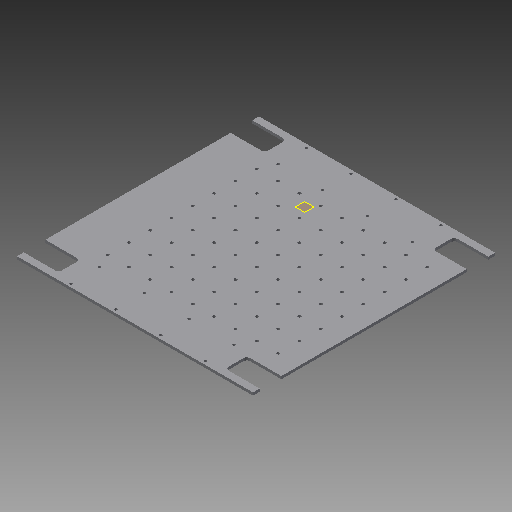
# Autodesk Inventor part: 1021TopP
Saved by Autodesk Inventor 2017 (Build 210142000, 142)
## iProperties
Created: 2016-09-29
Part Number: 1021TopP
Material: Generic
Document SubType Name: Modeling
Designer: Adam Popescu
Density: 1 g/cm^3
Appearance: Default
Author: Adam Popescu
Autodesk Inventor part; units mm, degrees
ref_plane "YZ Plane" through (0, 0, 0) normal (1, 0, 0) x (0, 1, 0)
ref_plane "XZ Plane" through (0, 0, 0) normal (0, 1, 0) x (-1, 0, 0)
ref_plane "XY Plane" through (0, 0, 0) normal (0, 0, 1) x (1, 0, 0)
sketch "Sketch1" plane through (0, 0, 0) normal (0, 1, 0) x (-1, 0, 0)
  circle A0 centre (-196.9946, -55.8186) radius 3.175
  circle A1 centre (-196.9946, -122.4936) radius 3.175
  circle A2 centre (-91.9021, -55.8186) radius 3.175
  circle A3 centre (13.1904, -55.8186) radius 3.175
  circle A4 centre (118.2829, -55.8186) radius 3.175
  circle A5 centre (-91.9021, -122.4936) radius 3.175
  circle A6 centre (13.1904, -122.4936) radius 3.175
  circle A7 centre (118.2829, -122.4936) radius 3.175
  line L0 (1428.2628, 61.5049) -> (1440.9628, 61.5049)
  line L1 (1966.4253, 57.5049) -> (1979.1253, 57.5049)
  circle A8 centre (-196.9946, 429.6364) radius 3.175
  circle A9 centre (-196.9946, 362.9614) radius 3.175
  circle A10 centre (-91.9021, 429.6364) radius 3.175
  circle A11 centre (13.1904, 429.6364) radius 3.175
  circle A12 centre (118.2829, 429.6364) radius 3.175
  circle A13 centre (-91.9021, 362.9614) radius 3.175
  circle A14 centre (13.1904, 362.9614) radius 3.175
  circle A15 centre (118.2829, 362.9614) radius 3.175
  line L2 (237.5784, -130.4286) -> (-316.2846, -130.4286)
  line L3 (-316.2846, -130.4286) -> (-316.2846, 437.5714)
  line L4 (-316.2846, 437.5714) -> (237.5784, 437.5714)
  line L5 (237.5784, 437.5714) -> (237.5784, -130.4286)
  line L6 (-236.5143, -106.5586) -> (-236.5143, -71.7586)
  arc A16 (-236.5143, -71.7586) -> (-244.5143, -63.7586) centre (-244.5143, -71.7586) ccw
  arc A17 (-244.5143, -114.5586) -> (-236.5143, -106.5586) centre (-244.5143, -106.5586) ccw
  line L7 (-244.5143, -63.7586) -> (-316.2846, -63.7586)
  line L8 (-244.5143, -114.5586) -> (-316.2846, -114.5586)
  line L9 (-235.2131, 378.9014) -> (-235.2131, 413.7014)
  arc A18 (-235.2131, 413.7014) -> (-243.2131, 421.7014) centre (-243.2131, 413.7014) ccw
  arc A19 (-243.2131, 370.9014) -> (-235.2131, 378.9014) centre (-243.2131, 378.9014) ccw
  line L10 (-243.2131, 421.7014) -> (-316.2846, 421.7014)
  line L11 (-243.2131, 370.9014) -> (-316.2846, 370.9014)
  line L12 (155.934, 378.9014) -> (155.934, 413.7014)
  arc A20 (163.934, 421.7014) -> (155.934, 413.7014) centre (163.934, 413.7014) ccw
  arc A21 (155.934, 378.9014) -> (163.934, 370.9014) centre (163.934, 378.9014) ccw
  line L13 (163.934, 421.7014) -> (237.5784, 421.7014)
  line L14 (163.934, 370.9014) -> (237.5784, 370.9014)
  line L15 (157.5215, -106.5586) -> (157.5215, -71.7586)
  line L16 (165.5215, -114.5586) -> (237.5784, -114.5586)
  line L17 (165.5215, -63.7586) -> (237.5784, -63.7586)
  arc A22 (165.5215, -63.7586) -> (157.5215, -71.7586) centre (165.5215, -71.7586) ccw
  arc A23 (157.5215, -106.5586) -> (165.5215, -114.5586) centre (165.5215, -106.5586) ccw
  point P0 (94.042, -85.1331)
  point P1 (-199.0181, 388.8507)
  point P2 (-236.5143, -63.7586)
  point P3 (-236.5143, -89.1586)
  point P4 (-235.2131, 421.7014)
  point P5 (-235.2131, 396.3014)
  dimension "d158" = 6.35
  dimension "d161" = 6.35
  dimension "d162" = 6.35
  dimension "d163" = 6.35
  dimension "d164" = 6.35
  dimension "d166" = 6.35
  dimension "d167" = 6.35
  dimension "d171" = 12.7
  dimension "d173" = 12.7
  dimension "d179" = 6.35
  dimension "d182" = 6.35
  dimension "d183" = 6.35
  dimension "d184" = 6.35
  dimension "d185" = 6.35
  dimension "d186" = 6.35
  dimension "d187" = 6.35
  dimension "d188" = 6.35
  dimension "d191" = 553.863
  dimension "d192" = 568
  dimension "d194" = 66.675
  dimension "d195" = 66.675
  dimension "d196" = 66.675
  dimension "d197" = 66.675
  dimension "d198" = 105.0925
  dimension "d199" = 105.0925
  dimension "d200" = 105.0925
  dimension "d201" = 105.0925
  dimension "d202" = 105.0925
  dimension "d203" = 105.0925
  dimension "d204" = 105.0925
  dimension "d205" = 66.675
  dimension "d206" = 66.675
  dimension "d207" = 66.675
  dimension "d318" = 15.87
  dimension "d319" = 7.935
  dimension "d320" = 15.87
  dimension "d321" = 7.935
  dimension "d324" = 15.87
  dimension "d325" = 15.87
  constraints: 36 end point, 24 centre point, 16 point on circle, 10 point on line, 4 tangent, 3 horizontal, 2 midpoint, 2 parallel, 1 perpendicular
  measures "d158" diameter of A0
  measures "d161" diameter of A2
  measures "d162" diameter of A1
  measures "d163" diameter of A5
  measures "d164" diameter of A3
  measures "d166" diameter of A4
  measures "d167" diameter of A7
  measures "d171" distance of L0.start L0.end
  measures "d173" distance of L1.start L1.end
  measures "d179" diameter of A8
  measures "d182" diameter of A10
  measures "d183" diameter of A9
  measures "d184" diameter of A13
  measures "d185" diameter of A11
  measures "d186" diameter of A14
  measures "d187" diameter of A12
  measures "d188" diameter of A15
  measures "d191" distance of L2.start L2.end
  measures "d192" distance of L4.end L2.start
  measures "d194" distance of A12.centre A15.centre
  measures "d195" distance of A11.centre A14.centre
  measures "d196" distance of A10.centre A13.centre
  measures "d197" distance of A8.centre A9.centre
  measures "d198" distance of A10.centre A8.centre
  measures "d199" distance of A11.centre A10.centre
  measures "d200" distance of A12.centre A11.centre
  measures "d201" distance of A3.centre A4.centre
  measures "d202" distance of A2.centre A3.centre
  measures "d203" distance of A0.centre A2.centre
  measures "d204" distance of A5.centre A1.centre
  measures "d205" distance of A1.centre A0.centre
  measures "d206" distance of A6.centre A3.centre
  measures "d207" distance of A4.centre A7.centre
  measures "d318" distance between parallel lines of L2 L8
  measures "d319" distance from line of L2 A6.centre
  measures "d320" distance between parallel lines of L4 L10
  measures "d321" distance from line of L4 A12.centre
  measures "d324" distance between parallel lines of L2 L16
  measures "d325" distance between parallel lines of L4 L13
ref_plane "Work Plane10" through (0, 6.35, 0) normal (0, 1, 0) x (1, 0, 0)
sketch "Sketch16" plane through (0, 6.35, 0) normal (0, 1, 0) x (1, 0, 0)
  circle A0 centre (-133.7154, 21.4286) radius 3.5
  circle A1 centre (-83.7154, 21.4286) radius 3.5
  circle A2 centre (-33.7154, 21.4286) radius 3.5
  circle A3 centre (16.2846, 21.4286) radius 3.5
  circle A4 centre (66.2846, 21.4286) radius 3.5
  circle A5 centre (116.2846, 21.4286) radius 3.5
  circle A6 centre (166.2846, 21.4286) radius 3.5
  circle A7 centre (216.2846, 21.4286) radius 3.5
  circle A8 centre (266.2846, 21.4286) radius 3.5
  circle A9 centre (-133.7154, -28.5714) radius 3.5
  circle A10 centre (-83.7154, -28.5714) radius 3.5
  circle A11 centre (-33.7154, -28.5714) radius 3.5
  circle A12 centre (16.2846, -28.5714) radius 3.5
  circle A13 centre (66.2846, -28.5714) radius 3.5
  circle A14 centre (116.2846, -28.5714) radius 3.5
  circle A15 centre (166.2846, -28.5714) radius 3.5
  circle A16 centre (216.2846, -28.5714) radius 3.5
  circle A17 centre (266.2846, -28.5714) radius 3.5
  circle A18 centre (-133.7154, -78.5714) radius 3.5
  circle A19 centre (-83.7154, -78.5714) radius 3.5
  circle A20 centre (-33.7154, -78.5714) radius 3.5
  circle A21 centre (16.2846, -78.5714) radius 3.5
  circle A22 centre (66.2846, -78.5714) radius 3.5
  circle A23 centre (116.2846, -78.5714) radius 3.5
  circle A24 centre (166.2846, -78.5714) radius 3.5
  circle A25 centre (216.2846, -78.5714) radius 3.5
  circle A26 centre (266.2846, -78.5714) radius 3.5
  circle A27 centre (-133.7154, -128.5714) radius 3.5
  circle A28 centre (-83.7154, -128.5714) radius 3.5
  circle A29 centre (-33.7154, -128.5714) radius 3.5
  circle A30 centre (16.2846, -128.5714) radius 3.5
  circle A31 centre (66.2846, -128.5714) radius 3.5
  circle A32 centre (116.2846, -128.5714) radius 3.5
  circle A33 centre (166.2846, -128.5714) radius 3.5
  circle A34 centre (216.2846, -128.5714) radius 3.5
  circle A35 centre (266.2846, -128.5714) radius 3.5
  circle A36 centre (-133.7154, -178.5714) radius 3.5
  circle A37 centre (-83.7154, -178.5714) radius 3.5
  circle A38 centre (-33.7154, -178.5714) radius 3.5
  circle A39 centre (16.2846, -178.5714) radius 3.5
  circle A40 centre (66.2846, -178.5714) radius 3.5
  circle A41 centre (116.2846, -178.5714) radius 3.5
  circle A42 centre (166.2846, -178.5714) radius 3.5
  circle A43 centre (216.2846, -178.5714) radius 3.5
  circle A44 centre (266.2846, -178.5714) radius 3.5
  circle A45 centre (-133.7154, -228.5714) radius 3.5
  circle A46 centre (-83.7154, -228.5714) radius 3.5
  circle A47 centre (-33.7154, -228.5714) radius 3.5
  circle A48 centre (16.2846, -228.5714) radius 3.5
  circle A49 centre (66.2846, -228.5714) radius 3.5
  circle A50 centre (116.2846, -228.5714) radius 3.5
  circle A51 centre (166.2846, -228.5714) radius 3.5
  circle A52 centre (216.2846, -228.5714) radius 3.5
  circle A53 centre (266.2846, -228.5714) radius 3.5
  circle A54 centre (-133.7154, -278.5714) radius 3.5
  circle A55 centre (-83.7154, -278.5714) radius 3.5
  circle A56 centre (-33.7154, -278.5714) radius 3.5
  circle A57 centre (16.2846, -278.5714) radius 3.5
  circle A58 centre (66.2846, -278.5714) radius 3.5
  circle A59 centre (116.2846, -278.5714) radius 3.5
  circle A60 centre (166.2846, -278.5714) radius 3.5
  circle A61 centre (216.2846, -278.5714) radius 3.5
  circle A62 centre (266.2846, -278.5714) radius 3.5
  circle A63 centre (-133.7154, -328.5714) radius 3.5
  circle A64 centre (-83.7154, -328.5714) radius 3.5
  circle A65 centre (-33.7154, -328.5714) radius 3.5
  circle A66 centre (16.2846, -328.5714) radius 3.5
  circle A67 centre (66.2846, -328.5714) radius 3.5
  circle A68 centre (116.2846, -328.5714) radius 3.5
  circle A69 centre (166.2846, -328.5714) radius 3.5
  circle A70 centre (216.2846, -328.5714) radius 3.5
  circle A71 centre (266.2846, -328.5714) radius 3.5
  line L0 (-237.5784, 130.4286) -> (316.2846, 130.4286) projected
  line L1 (-237.5784, -437.5714) -> (316.2846, -437.5714) projected
  line L2 (-237.5784, 130.4286) -> (-237.5784, -437.5714) projected
  line L3 (316.2846, -437.5714) -> (316.2846, 130.4286) projected
  dimension "d220" = 7
  dimension "d221" = 50
  dimension "d222" = 50
  dimension "d225" = 50
  dimension "d226" = 50
  dimension "d227" = 50
  dimension "d228" = 50
  dimension "d229" = 50
  dimension "d230" = 50
  dimension "d231" = 50
  dimension "d232" = 50
  dimension "d233" = 50
  dimension "d234" = 50
  dimension "d235" = 50
  dimension "d236" = 50
  dimension "d237" = 50
  dimension "d238" = 50
  dimension "d239" = 50
  dimension "d240" = 50
  dimension "d241" = 50
  dimension "d242" = 50
  dimension "d243" = 50
  dimension "d244" = 50
  dimension "d245" = 50
  dimension "d246" = 50
  dimension "d247" = 50
  dimension "d248" = 50
  dimension "d249" = 50
  dimension "d250" = 50
  dimension "d251" = 50
  dimension "d252" = 50
  dimension "d253" = 50
  dimension "d254" = 50
  dimension "d255" = 50
  dimension "d256" = 50
  dimension "d257" = 50
  dimension "d258" = 50
  dimension "d259" = 50
  dimension "d260" = 50
  dimension "d261" = 50
  dimension "d262" = 50
  dimension "d263" = 50
  dimension "d264" = 50
  dimension "d265" = 50
  dimension "d266" = 50
  dimension "d267" = 50
  dimension "d268" = 50
  dimension "d269" = 50
  dimension "d270" = 50
  dimension "d271" = 50
  dimension "d272" = 50
  dimension "d273" = 50
  dimension "d274" = 50
  dimension "d275" = 50
  dimension "d276" = 50
  dimension "d277" = 50
  dimension "d278" = 50
  dimension "d279" = 50
  dimension "d280" = 50
  dimension "d281" = 50
  dimension "d282" = 50
  dimension "d283" = 50
  dimension "d284" = 50
  dimension "d285" = 50
  constraints: 72 centre point
  measures "d220" diameter of A0
  measures "d221" distance of A0.centre A1.centre
  measures "d222" distance of A0.centre A9.centre
  measures "d225" distance of A2.centre A1.centre
  measures "d226" distance of A3.centre A2.centre
  measures "d227" distance of A4.centre A3.centre
  measures "d228" distance of A5.centre A4.centre
  measures "d229" distance of A6.centre A5.centre
  measures "d230" distance of A7.centre A6.centre
  measures "d231" distance of A8.centre A7.centre
  measures "d232" distance of A17.centre A8.centre
  measures "d233" distance of A26.centre A17.centre
  measures "d234" distance of A26.centre A35.centre
  measures "d235" distance of A35.centre A44.centre
  measures "d236" distance of A44.centre A53.centre
  measures "d237" distance of A53.centre A62.centre
  measures "d238" distance of A62.centre A71.centre
  measures "d239" distance of A70.centre A71.centre
  measures "d240" distance of A61.centre A62.centre
  measures "d241" distance of A60.centre A61.centre
  measures "d242" distance of A69.centre A70.centre
  measures "d243" distance of A68.centre A69.centre
  measures "d244" distance of A67.centre A68.centre
  measures "d245" distance of A66.centre A67.centre
  measures "d246" distance of A65.centre A66.centre
  measures "d247" distance of A64.centre A65.centre
  measures "d248" distance of A63.centre A64.centre
  measures "d249" distance of A59.centre A60.centre
  measures "d250" distance of A58.centre A59.centre
  measures "d251" distance of A57.centre A58.centre
  measures "d252" distance of A56.centre A57.centre
  measures "d253" distance of A55.centre A56.centre
  measures "d254" distance of A54.centre A55.centre
  measures "d255" distance of A46.centre A45.centre
  measures "d256" distance of A46.centre A47.centre
  measures "d257" distance of A48.centre A47.centre
  measures "d258" distance of A48.centre A49.centre
  measures "d259" distance of A49.centre A50.centre
  measures "d260" distance of A50.centre A51.centre
  measures "d261" distance of A51.centre A52.centre
  measures "d262" distance of A52.centre A53.centre
  measures "d263" distance of A10.centre A9.centre
  measures "d264" distance of A11.centre A10.centre
  measures "d265" distance of A12.centre A11.centre
  measures "d266" distance of A13.centre A12.centre
  measures "d267" distance of A14.centre A13.centre
  measures "d268" distance of A15.centre A14.centre
  measures "d269" distance of A16.centre A15.centre
  measures "d270" distance of A24.centre A25.centre
  measures "d271" distance of A23.centre A24.centre
  measures "d272" distance of A34.centre A25.centre
  measures "d273" distance of A43.centre A34.centre
  measures "d274" distance of A33.centre A34.centre
  measures "d275" distance of A42.centre A43.centre
  measures "d276" distance of A33.centre A32.centre
  measures "d277" distance of A41.centre A42.centre
  measures "d278" distance of A50.centre A41.centre
  measures "d279" distance of A40.centre A31.centre
  measures "d280" distance of A30.centre A21.centre
  measures "d281" distance of A40.centre A39.centre
  measures "d282" distance of A23.centre A22.centre
  measures "d283" distance of A30.centre A31.centre
  measures "d284" distance of A48.centre A39.centre
  measures "d285" distance of A29.centre A20.centre
extrude "Extrusion11" add sketch "Sketch1" along normal blind 6.35 contours L2 L3 L8 A17 L6 A16 L7 L11 A19 L9 A18 L10 L4 L5 L13 A20 L12 A21 L14 L17 A22 L15 A23 L16
hole "Hole3" at (-83.7154, 6.35, 178.5714) at (-133.7154, 6.35, 228.5714) at (266.2846, 6.35, 178.5714) at (166.2846, 6.35, 178.5714) at (-133.7154, 6.35, 28.5714) at (-133.7154, 6.35, 128.5714) at (-133.7154, 6.35, 78.5714) at (-33.7154, 6.35, 128.5714) at (16.2846, 6.35, 128.5714) at (16.2846, 6.35, 178.5714) at (266.2846, 6.35, 228.5714) at (-33.7154, 6.35, 178.5714) at (66.2846, 6.35, 128.5714) at (66.2846, 6.35, 178.5714) at (116.2846, 6.35, 178.5714) at (166.2846, 6.35, 128.5714) at (216.2846, 6.35, 178.5714) at (216.2846, 6.35, 128.5714) at (116.2846, 6.35, 128.5714) at (216.2846, 6.35, 228.5714) at (166.2846, 6.35, 228.5714) at (116.2846, 6.35, 228.5714) at (66.2846, 6.35, 228.5714) at (116.2846, 6.35, 278.5714) at (66.2846, 6.35, 278.5714) at (166.2846, 6.35, 328.5714) at (116.2846, 6.35, 328.5714) at (66.2846, 6.35, 328.5714) at (-83.7154, 6.35, 128.5714) at (-33.7154, 6.35, 278.5714) at (-133.7154, 6.35, 178.5714) at (-33.7154, 6.35, 328.5714) at (-83.7154, 6.35, 278.5714) at (-133.7154, 6.35, 278.5714) at (-83.7154, 6.35, 228.5714) at (-33.7154, 6.35, 228.5714) at (16.2846, 6.35, 278.5714) at (16.2846, 6.35, 228.5714) at (-133.7154, 6.35, 328.5714) at (116.2846, 6.35, 28.5714) at (116.2846, 6.35, -21.4286) at (216.2846, 6.35, 28.5714) at (216.2846, 6.35, 78.5714) at (266.2846, 6.35, 78.5714) at (116.2846, 6.35, 78.5714) at (66.2846, 6.35, 28.5714) at (166.2846, 6.35, 28.5714) at (216.2846, 6.35, -21.4286) at (266.2846, 6.35, -21.4286) at (166.2846, 6.35, -21.4286) direction (0, -1, 0) diameter 7 end through all and at (166.2846, 6.35, 78.5714) (266.2846, 6.35, 28.5714) (266.2846, 6.35, 128.5714) (266.2846, 6.35, 328.5714) (216.2846, 6.35, 328.5714) (266.2846, 6.35, 278.5714) (216.2846, 6.35, 278.5714) (166.2846, 6.35, 278.5714) (-83.7154, 6.35, 328.5714) (16.2846, 6.35, 328.5714) (-83.7154, 6.35, 78.5714) (-33.7154, 6.35, 28.5714) (16.2846, 6.35, -21.4286) (-33.7154, 6.35, -21.4286) (66.2846, 6.35, -21.4286) (16.2846, 6.35, 28.5714) (-83.7154, 6.35, -21.4286) (16.2846, 6.35, 78.5714) (-83.7154, 6.35, 28.5714) (-33.7154, 6.35, 78.5714) (-133.7154, 6.35, -21.4286) (66.2846, 6.35, 78.5714)
body "Solid1"
